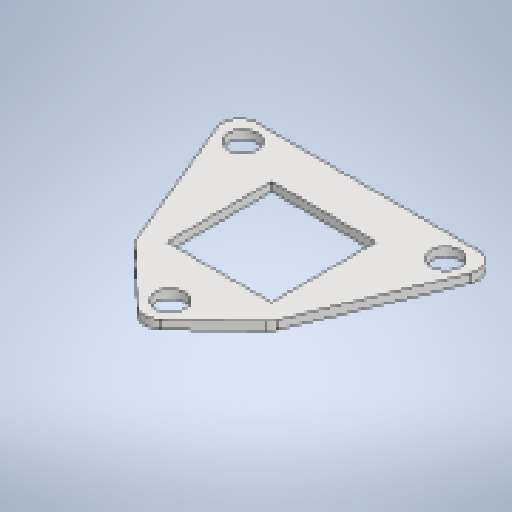
# Autodesk Inventor part: DS-B-501 beam flange
Saved by Autodesk Inventor 2025 (Build 290162010, 162A)
## iProperties
Created: 2025-01-13
Part Number: DS-B-501 beam flange
Material: Stainless Steel
Document SubType Name: Sheet Metal
Designer: user
Mass: 280.619 g
Surface Area: 364.406 cm^2
Volume: 35.0774 cm^3
Density: 8 g/cm^3
Sheet Metal Rule: AISI304 3mm Die 32
Sheet Metal Width: 76,751 mm
Sheet Metal Length: 87,968 mm
Sheet Metal Area: 6751,660 mm^2
Appearance: Default
Flat Pattern Width: 7.67513 cm
Flat Pattern Length: 8.7968 cm
Flat Pattern Area: 67.5166 cm^2
Author: user
Autodesk Inventor part; units mm, degrees
ref_plane "YZ Plane" through (0, 0, 0) normal (1, 0, 0) x (0, 1, 0)
ref_plane "XZ Plane" through (0, 0, 0) normal (0, 1, 0) x (-1, 0, 0)
ref_plane "XY Plane" through (0, 0, 0) normal (0, 0, 1) x (1, 0, 0)
sketch "Sketch6" plane through (0, 0, 0) normal (0, 0, 1) x (1, 0, 0)
  line L0 (18, 18) -> (-18, 18)
  line L1 (-18, 18) -> (-18, -18)
  line L2 (-18, -18) -> (18, -18)
  line L3 (18, -18) -> (18, 18)
  line L4 (18, 18) -> (-18, -18) construction
  circle A0 centre (0, -35) radius 5.05
  circle A1 centre (35, 25) radius 5.05
  circle A2 centre (-35, 25) radius 5.05
  line L5 (35, 25) -> (-35, 25) construction
  line L6 (-35, 25) -> (0, -35) construction
  line L7 (0, -35) -> (35, 25) construction
  line L8 (0, 18) -> (0, -18) construction
  line L9 (-46.936, 33) -> (46.936, 33)
  line L10 (-18, 18) -> (23.6569, -23.6569) construction
  line L11 (18, 18) -> (-23.6569, -23.6569) construction
  line L12 (46.936, 33) -> (23.6569, -23.6569)
  line L13 (23.6569, -23.6569) -> (0, -46.0053)
  line L14 (0, -46.0053) -> (-23.6569, -23.6569)
  line L15 (-46.936, 33) -> (-23.6569, -23.6569)
  line L16 (-35, 25) -> (-42.3997, 21.9596) construction
  line L17 (0, -35) -> (-5.4937, -40.8154) construction
  point P0 (0, 0)
  point P1 (0, 0)
  point P2 (60, 0)
  point P3 (0, 33)
  point P4 (0, 0)
  dimension "d30" = 36
  dimension "d31" = 36
  dimension "d33" = 10.1
  dimension "d37" = 69.4622
  dimension "d52" = 70
  dimension "d53" = 8
  dimension "d54" = 25
  dimension "d57" = 8
  dimension "d59" = 8
  dimension "d60" = 93.872
  dimension "d61" = 60
  dimension "d62" = 8
  dimension "d63" = 8
  measures "d30" distance of L2.end L1.end
  measures "d31" distance of L1.end L1.start
  measures "d33" diameter of A0
  measures "d37" distance of L6.start L6.end
  measures "d52" distance of L5.start L6.start
  measures "d53" distance between parallel lines of L5 L9
  measures "d54" distance from line of point (0, 0) L5
  measures "d57" distance of L11.end L1.end
  measures "d59" distance of L10.end L2.end
  measures "d60" distance of L9.start L9.end
  measures "d61" distance from line of L6.end L5
  measures "d62" distance of L6.start L16.end
  measures "d63" distance of L6.end L17.end
extrude "Plate3" add sketch "Sketch6" along normal blind 3
fillet "Corner Round2" radius 6 5 edges at (-46.936, 33, 1.5) (46.936, 33, 1.5) (0, -46.0053, 1.5) (-23.6569, -23.6569, 1.5) (23.6569, -23.6569, 1.5)
equation "\"d41\" = Thickness"
equation "\"BendReliefWidth\" = Thickness"
equation "\"BendReliefDepth\" = 0.5 * Thickness"
equation "\"CornerReliefSize\" = 4 * Thickness"
equation "\"MinimumRemnant\" = 2 * Thickness"
equation "\"TransitionRadius\" = BendRadius"
equation "\"JacobiRadiusSize\" = BendRadius"
equation "\"GapSize\" = Thickness"
equation "\"Thickness\" = 3"
equation "\"BendRadius\" = 5"
body "Solid2"
